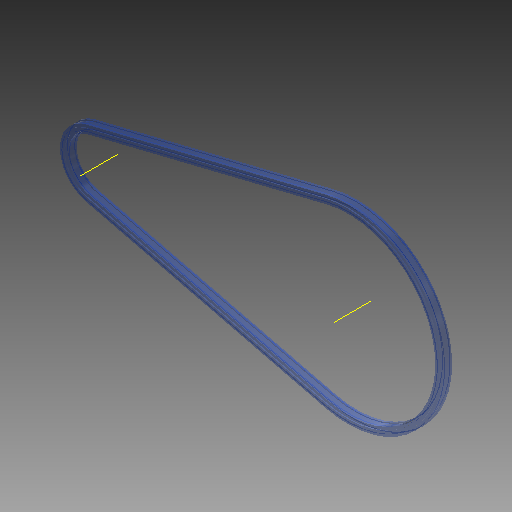
# Autodesk Inventor part: Rollenkette
Saved by Autodesk Inventor 2018 (Build 220112000, 112)
## iProperties
Created: 2018-01-11
Part Number: Rollenkette
Material: Generic
Document SubType Name: Modeling
Designer: Dominik
Density: 1 g/cm^3
Appearance: Clear - Blue
CustomPartVersion: 1
Author: Dominik
Autodesk Inventor part; units mm, degrees
ref_plane "Arbeitsebene2" through (-120.9582, 0, 0) normal (-1, 0, 0) x (0, 0, 1)
ref_plane "Arbeitsebene3" through (200, 0, 0) normal (-0.9757842, -0.2187353, 0) x (0, 0, 1)
sketch "Pfad" plane through (0, 0, 0) normal (0, 0, 1) x (1, 0, 0)
  arc A0 (-130.1766, 37.4621) -> (-130.1766, -37.4621) centre (-120.9582, 0) ccw
  arc A1 (172.4568, -111.9316) -> (172.4568, 111.9316) centre (200, 0) ccw
  line L0 (172.4568, -111.9316) -> (-130.1766, -37.4621)
  line L1 (-130.1766, 37.4621) -> (172.4568, 111.9316)
  dimension "d31" = 9.91
  constraints: 4 end point, 4 point on circle, 2 centre point
ref_plane "Profilebene" through (-130.1766, -37.4621, 0) normal (0.9710334, -0.2389438, 0) x (0, 0, 1)
sketch "Profilskizze" plane through (-130.1766, -37.4621, 0) normal (0.9710334, -0.2389438, 0) x (0, 0, 1)
  line L0 (-7, -1.8) -> (7, -1.8)
  line L1 (7, -1.8) -> (7, 1.8)
  line L2 (7, 1.8) -> (-7, 1.8)
  line L3 (-7, 1.8) -> (-7, -1.8)
  line L4 (-3.125, -3.885) -> (3.125, -3.885)
  line L5 (3.125, -3.885) -> (3.125, 3.885)
  line L6 (3.125, 3.885) -> (-3.125, 3.885)
  line L7 (-3.125, 3.885) -> (-3.125, -3.885)
  line L8 (-3.125, 0) -> (3.125, 0) construction
  line L9 (-5.725, -4.955) -> (-3.125, -4.955)
  line L10 (-3.125, -4.955) -> (-3.125, 4.955)
  line L11 (-3.125, 4.955) -> (-5.725, 4.955)
  line L12 (-5.725, 4.955) -> (-5.725, -4.955)
  line L13 (3.125, -4.955) -> (5.725, -4.955)
  line L14 (5.725, -4.955) -> (5.725, 4.955)
  line L15 (5.725, 4.955) -> (3.125, 4.955)
  line L16 (3.125, 4.955) -> (3.125, -4.955)
  line L17 (-7, 0) -> (7, 0) construction
  point P0 (0, 0)
  point P1 (0, 0)
  dimension "d21" = 3.6
  dimension "d22" = 7.77
  dimension "d23" = 6.25
  dimension "d24" = 2.6
  dimension "d31" = 9.91
  dimension "d32" = 14
  constraints: 36 end point, 8 midpoint, 8 parallel, 4 horizontal, 4 perpendicular, 3 collinear, 1 coincident, 1 other
  measures "d21" distance between parallel lines of L2 L0
  measures "d22" distance between parallel lines of L6 L4
  measures "d23" distance between parallel lines of L5 L7
  measures "d24" distance between parallel lines of L12 L10
  measures "d31" distance between parallel lines of L11 L9
  measures "d32" distance between parallel lines of L1 L3
sweep "Volumenkörper" add profiles "Profilskizze" path "Pfad"
pattern_of_one "Strand Pattern"
equation "\"d21\" = da_d2"
equation "\"d22\" = da_d1"
equation "\"d23\" = da_b1"
equation "\"d24\" = da_t1 + da_t2"
equation "\"d30\" = da_pt"
equation "\"da_p\" = 12.7"
equation "\"da_b1\" = 6.25"
equation "\"da_h2\" = 9.91"
equation "\"da_h3\" = 8.51"
equation "\"da_d1\" = 7.77"
equation "\"da_d2\" = 3.6"
equation "\"da_pt\" = 13.92"
equation "\"da_b\" = 14"
equation "\"da_t1\" = 1.3"
equation "\"da_t2\" = 1.3"
body "Solid1"
